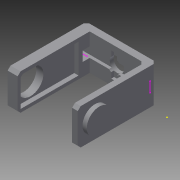
# Autodesk Inventor part: Enlace2Base
Saved by Autodesk Inventor 2014 SP1 (Build 180222100, 222)
## iProperties
Created: 2013-10-22
Part Number: Enlace2Base
Material: Genérico
Document SubType Name: Modeling
Designer: Gregorio
Density: 1 g/cm^3
Appearance: Valor por defecto
Author: Gregorio
Autodesk Inventor part; units mm, degrees
ref_plane "YZ Plane" through (0, 0, 0) normal (1, 0, 0) x (0, 1, 0)
ref_plane "XZ Plane" through (0, 0, 0) normal (0, 1, 0) x (-1, 0, 0)
ref_plane "XY Plane" through (0, 0, 0) normal (0, 0, 1) x (1, 0, 0)
sketch "Boceto1" plane through (0, 0, 0) normal (0, 0, 1) x (1, 0, 0)
  line L0 (-12, 0) -> (-16, 0)
  line L1 (-16, 0) -> (-16, 55)
  line L2 (-16, 55) -> (-12, 55)
  line L3 (-12, 55) -> (-12, 0)
  line L4 (-12, 55) -> (-62, 55)
  line L5 (-62, 55) -> (-62, 50.3)
  line L6 (-62, 50.3) -> (-12, 50.3)
  line L7 (-12, 50.3) -> (-12, 55)
  line L8 (-62, 55) -> (-58, 55)
  line L9 (-58, 55) -> (-58, 0)
  line L10 (-58, 0) -> (-62, 0)
  line L11 (-62, 0) -> (-62, 55)
  dimension "d4" = 4
  dimension "d5" = 55
  dimension "d6" = 50
  dimension "d7" = 4.7
  dimension "d8" = 4
  dimension "d9" = 55
  constraints: 24 end point, 6 parallel, 3 horizontal, 3 perpendicular
  measures "d4" distance of L1.end L2.end
  measures "d5" distance of L0.end L1.end
  measures "d6" distance of L6.end L5.end
  measures "d7" distance of L5.end L4.end
  measures "d8" distance of L9.end L10.end
  measures "d9" distance of L8.end L9.end
extrude "Extrusión1" add sketch "Boceto1" along normal blind 25
sketch "Boceto2" plane through (-58, 0, 0) normal (1, 0, 0) x (0, 0, -1)
  line L0 (-25, 0) -> (-25, 50.3) projected
  circle A0 centre (-12.5, 12) radius 9
  line L1 (0, 0) -> (-25, 0) projected
  dimension "d12" = 12.5
  dimension "d13" = 18
  dimension "d21" = 12
  constraints: 1 centre point
  measures "d12" distance from line of L0 A0.centre
  measures "d13" diameter of A0
  measures "d21" distance from line of L1 A0.centre
extrude "Extrusión2" cut sketch "Boceto2" against normal blind 15
sketch "Boceto3" plane through (-12, 0, 0) normal (1, 0, 0) x (0, 0, -1)
  line L0 (0, 0) -> (0, 55) projected
  line L1 (0, 0) -> (-25, 0) projected
  circle A0 centre (-12.5, 12) radius 8.75
  dimension "d16" = 17.5
  dimension "d17" = 12
  dimension "d18" = 12.5
  constraints: 1 centre point
  measures "d16" diameter of A0
  measures "d17" distance from line of L1 A0.centre
  measures "d18" distance from line of L0 A0.centre
extrude "Extrusión3" add sketch "Boceto3" along normal blind 3
sketch "Boceto4" plane through (-58, 0, 0) normal (1, 0, 0) x (0, 0, -1)
  circle A0 centre (-12.5, 12) radius 9 projected
  line L0 (0, 50.3) -> (-25, 50.3) projected
  line L1 (-25, 0) -> (-25, 50.3) projected
  line L2 (0, 0) -> (-25, 0) projected
  line L3 (0, 0) -> (0, 50.3) projected
extrude "Extrusión4" add sketch "Boceto4" along normal blind 4
sketch "Boceto7" plane through (-62, 55, 0) normal (0, 1, 0) x (1, 0, 0)
  line L0 (50, 0) -> (0, 0)
  circle A0 centre (25, -12.5) radius 5
  line L1 (6.5, -9) -> (43.5, -9)
  line L2 (43.5, -9) -> (43.5, -16)
  line L3 (43.5, -16) -> (6.5, -16)
  line L4 (6.5, -16) -> (6.5, -9)
  line L5 (23, -4) -> (27, -4)
  line L6 (27, -4) -> (27, -21)
  line L7 (27, -21) -> (23, -21)
  line L8 (23, -21) -> (23, -4)
  line L9 (50, 0) -> (0, 0) projected
  point P0 (58, 0)
  point P1 (6.5, -12.5)
  point P2 (25, -9)
  point P3 (23, -12.5)
  point P4 (25, -4)
  point P5 (25, 0)
  dimension "d29" = 10
  dimension "d30" = 37
  dimension "d31" = 7
  dimension "d32" = 12.5
  dimension "d33" = 4
  dimension "d34" = 17
  constraints: 18 end point, 5 midpoint, 4 parallel, 3 vertical alignment, 2 horizontal, 2 horizontal alignment, 2 perpendicular, 1 centre point
  measures "d29" diameter of A0
  measures "d30" distance of L2.end L3.end
  measures "d31" distance of L3.end L1.start
  measures "d32" distance from line of L0 A0.centre
  measures "d33" distance of L6.end L7.end
  measures "d34" distance of L7.end L5.start
extrude "Extrusión6" cut sketch "Boceto7" against normal blind 10 contours A0 L3 L6 L1 | L1 L6 A0 | A0 L6 L3 | L6 L1 L8 A0 | L6 L3 L8 L1 | A0 L8 L3 L6 | L8 L1 A0 | L8 L3 A0 L1 | A0 L3 L8
sketch "Boceto8" plane through (-16, 50.3, 0) normal (0, -1, 0) x (1, 0, 0)
  line L0 (-39.5, 9) -> (-2.5, 9) projected
  line L1 (-39.5, 16) -> (-39.5, 9) projected
  line L2 (-2.5, 16) -> (-39.5, 16) projected
  line L3 (-2.5, 9) -> (-2.5, 16) projected
  circle A0 centre (-21, 12.5) radius 5 projected
  line L4 (-23, 21) -> (-23, 4) projected
  line L5 (-23, 4) -> (-19, 4) projected
  line L6 (-19, 4) -> (-19, 21) projected
  line L7 (-19, 21) -> (-23, 21) projected
  point P0 (16, 0)
extrude "Extrusión8" cut sketch "Boceto8" against normal blind 2 contours L1 L2 A0 L0 | A0 L2 L4 L0 | L4 L2 L6 L0 | L6 L2 A0 L0 | A0 L2 L3 L0
sketch "Boceto9" plane through (-16, 50.3, 0) normal (0, -1, 0) x (1, 0, 0)
  line L0 (-19, 4) -> (-19, 21) projected
  line L1 (-23, 21) -> (-23, 4) projected
  line L2 (-23, 4) -> (-19, 4) projected
  line L3 (-19, 21) -> (-23, 21) projected
  point P0 (16, 0)
extrude "Extrusión9" cut sketch "Boceto9" against normal blind 2
sketch "Boceto10" plane through (-54, 0, 0) normal (1, 0, 0) x (0, 0, -1)
  line L0 (-16, 50.3) -> (-9, 50.3)
  line L1 (-9, 50.3) -> (-9, 48.8686)
  line L2 (-9, 48.8686) -> (-16, 48.8686)
  line L3 (-16, 48.8686) -> (-16, 50.3)
  dimension "d43" = 7
  dimension "d44" = 1.4314
  constraints: 8 end point, 2 parallel, 1 horizontal, 1 perpendicular
  measures "d43" distance of L1.end L2.end
  measures "d44" distance of L0.end L1.end
extrude "Extrusión10" cut sketch "Boceto10" against normal blind 2
chamfer "Chaflán3" distance 2 angle 45 1 edges at (-16, 50.3, 12.5)
chamfer "Chaflán4" distance 2 angle 45 1 edges at (-12, 55, 12.5)
sketch "Boceto11" plane through (-16, 50.3, 0) normal (0, 1, 0) x (1, 0, 0)
  line L0 (2, -16) -> (2, -9) projected
  line L1 (-40, -16) -> (-43.5, -16) projected
  line L2 (4, -9) -> (4, -16) projected
  line L3 (-43.5, -9) -> (-40, -9) projected
  point P0 (16, 0)
sketch "Boceto14" plane through (-62, 0, 0) normal (-1, 0, 0) x (0, 0, 1)
  circle A0 centre (12.5, 12) radius 9 projected
  line L0 (25, 55) -> (25, 0) projected
  line L1 (0, 55) -> (25, 55) projected
  line L2 (0, 55) -> (0, 0) projected
  line L3 (0, 0) -> (25, 0) projected
  circle A1 centre (12.5, 12) radius 10
  constraints: 1 centre point, 1 coincident
extrude "Extrusión13" cut sketch "Boceto14" against normal blind 1 contours L0 L3 L2 L1
chamfer "Chaflán8" distance 2 angle 45 1 edges at (-61, 55, 12.5)
chamfer "Chaflán10" distance 2 angle 45 4 edges at (-57.5, 0, 0) (-57.5, 0, 25) (-14, 0, 25) (-14, 0, 0)
sketch "Boceto18" plane through (-54, 0, 0) normal (1, 0, 0) x (0, 0, -1)
  line L0 (-16, 50.3) -> (-9, 50.3)
  line L1 (-9, 50.3) -> (-9, 45.3)
  line L2 (-9, 45.3) -> (-16, 45.3)
  line L3 (-16, 45.3) -> (-16, 50.3)
  point P0 (0, 0)
  constraints: 8 end point, 2 parallel, 1 horizontal, 1 perpendicular
extrude "Extrusión17" cut sketch "Boceto18" against normal blind 10
sketch "Boceto19" plane through (-55.5, 52.3, 16) normal (1, 0, 0) x (0, 0, -1)
  line L0 (0, -2) -> (7, -2) projected
  line L1 (7, -2) -> (7, 0) projected
  line L2 (7, 0) -> (0, 0) projected
  line L3 (0, -2) -> (0, 0) projected
  point P0 (16, -52.3)
extrude "Extrusión18" cut sketch "Boceto19" against normal blind 10
sketch "Boceto20" plane through (-54, 0, 0) normal (1, 0, 0) x (0, 0, -1)
  line L0 (-25, 50.3) -> (-16, 50.3) projected
  circle A0 centre (-12.5, 12) radius 9 projected
  line L1 (-22.75, 42.5) -> (-2.25, 42.5)
  line L2 (-2.25, 42.5) -> (-2.25, 2)
  line L3 (-2.25, 2) -> (-22.75, 2)
  line L4 (-22.75, 2) -> (-22.75, 42.5)
  line L5 (-22.75, 42.5) -> (-2.25, 2) construction
  line L6 (-2.25, 42.5) -> (-22.75, 2) construction
  line L7 (-22.75, 42.5) -> (-2.25, 42.5) construction
  point P0 (0, 0)
  point P1 (-12.5, 22.25)
  point P2 (-12.5, 2)
  dimension "d100" = 20.5
  dimension "d102" = 40.5
  dimension "d103" = 10
  constraints: 14 end point, 3 midpoint, 3 parallel, 1 collinear, 1 horizontal, 1 perpendicular, 1 vertical alignment
  measures "d100" distance of L1.start L1.end
  measures "d102" distance of L1.end L2.end
  measures "d103" distance from line of L3 A0.centre
extrude "Extrusión19" cut sketch "Boceto20" against normal blind 3
